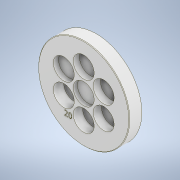
# Autodesk Inventor part: Diameter_20mm
Saved by Autodesk Inventor 2021 (Build 250183000, 183)
## iProperties
Created: 2023-09-28
Part Number: Diameter_20mm
Material: Polypropylen
Document SubType Name: Modeling
Designer: Konstantin
Density: 0.899 g/cm^3
Appearance: Glatt - Esche
Author: Konstantin
Autodesk Inventor part; units mm, degrees
ref_plane "YZ Plane" through (0, 0, 0) normal (1, 0, 0) x (0, 1, 0)
ref_plane "XZ Plane" through (0, 0, 0) normal (0, 1, 0) x (-1, 0, 0)
ref_plane "XY Plane" through (0, 0, 0) normal (0, 0, 1) x (1, 0, 0)
sketch "Sketch1" plane through (0, 0, 0) normal (0, 0, 1) x (1, 0, 0)
  circle A0 centre (0, 0) radius 43.5
  circle A1 centre (0, 0) radius 10
  circle A2 centre (0, 22) radius 10
  circle A3 centre (-19.0526, 11) radius 10
  circle A4 centre (-19.0526, -11) radius 10
  circle A5 centre (0, -22) radius 10
  circle A6 centre (19.0526, -11) radius 10
  circle A7 centre (19.0526, 11) radius 10
  dimension "diameter" = 20
  dimension "d2" = 20
  dimension "d5" = 360
  dimension "d7" = 22
  dimension "d28" = 87
  constraints: 8 centre point, 2 coincident, 13 other
  measures "diameter" diameter of A1
  measures "d2" diameter of A2
  measures "d7" distance of point (0, 0) A2.centre
  measures "d28" diameter of A0
extrude "Extrusion1" add sketch "Sketch1" along normal blind 12
sketch "Sketch2" plane through (0, 0, 12) normal (0, 0, 1) x (1, 0, 0)
  line L0 (-5.8774, 39.105) -> (5.7366, 39.105) construction
  line L1 (5.7366, 39.105) -> (5.7366, 35.936) construction
  line L2 (5.7366, 35.936) -> (-5.8774, 35.936) construction
  line L3 (-5.8774, 35.936) -> (-5.8774, 39.105) construction
  point P0 (0, 0)
  constraints: 2 other
emboss "Emboss1" [suppressed]
chamfer "Chamfer1" distance 0.5 angle 45 1 edges at (-43.5, 0, 12)
extrude "Extrusion11" add sketch "Sketch1" along normal blind 2 contours A4
extrude "Extrusion12" add sketch "Sketch1" along normal blind 3 contours A5
extrude "Extrusion13" add sketch "Sketch1" along normal blind 4 contours A6
extrude "Extrusion14" add sketch "Sketch1" along normal blind 5 contours A7
extrude "Extrusion15" add sketch "Sketch1" along normal blind 6 contours A2
extrude "Extrusion16" add sketch "Sketch1" along normal blind 7 contours A3
extrude "Extrusion17" add sketch "Sketch1" along normal blind 8 contours A1
sketch "Skizze3" plane through (0, 0, 12) normal (0, 0, 1) x (1, 0, 0)
  line L0 (-4.3129, -31.1582) -> (0.2616, -31.1582) construction
  line L1 (0.2616, -31.1582) -> (0.2616, -34.3322) construction
  line L2 (0.2616, -34.3322) -> (-4.3129, -34.3322) construction
  line L3 (-4.3129, -34.3322) -> (-4.3129, -31.1582) construction
  line L4 (28.3417, 16.1952) -> (30.6289, 16.1952) construction
  line L5 (30.6289, 16.1952) -> (30.6289, 13.0262) construction
  line L6 (30.6289, 13.0262) -> (28.3417, 13.0262) construction
  line L7 (28.3417, 13.0262) -> (28.3417, 16.1952) construction
  line L8 (-27.2854, 19.1878) -> (-24.9982, 19.1878) construction
  line L9 (-24.9982, 19.1878) -> (-24.9982, 16.0015) construction
  line L10 (-24.9982, 16.0015) -> (-27.2854, 16.0015) construction
  line L11 (-27.2854, 16.0015) -> (-27.2854, 19.1878) construction
  line L12 (-18.5838, -22.0358) -> (-14.0094, -22.0358) construction
  line L13 (-14.0094, -22.0358) -> (-14.0094, -25.2048) construction
  line L14 (-14.0094, -25.2048) -> (-18.5838, -25.2048) construction
  line L15 (-18.5838, -25.2048) -> (-18.5838, -22.0358) construction
  line L16 (-11.1833, -16.7575) -> (-8.896, -16.7575) construction
  line L17 (-8.896, -16.7575) -> (-8.896, -19.8055) construction
  line L18 (-8.896, -19.8055) -> (-11.1833, -19.8055) construction
  line L19 (-11.1833, -19.8055) -> (-11.1833, -16.7575) construction
  line L20 (20.4292, 1.4865) -> (22.7164, 1.4865) construction
  line L21 (22.7164, 1.4865) -> (22.7164, -1.6825) construction
  line L22 (22.7164, -1.6825) -> (20.4292, -1.6825) construction
  line L23 (20.4292, -1.6825) -> (20.4292, 1.4865) construction
  line L24 (-11.5764, 19.8878) -> (-9.2892, 19.8878) construction
  line L25 (-9.2892, 19.8878) -> (-9.2892, 16.7756) construction
  line L26 (-9.2892, 16.7756) -> (-11.5764, 16.7756) construction
  line L27 (-11.5764, 16.7756) -> (-11.5764, 19.8878) construction
  line L28 (3.9152, 10.1367) -> (6.2025, 10.1367) construction
  line L29 (6.2025, 10.1367) -> (6.2025, 7.0887) construction
  line L30 (6.2025, 7.0887) -> (3.9152, 7.0887) construction
  line L31 (3.9152, 7.0887) -> (3.9152, 10.1367) construction
  line L32 (-15.1357, -27.1411) -> (-18.2192, -27.1411)
  line L33 (-18.2192, -27.1411) -> (-18.2192, -26.432)
  spline S0 degree 2 poles (-18.2192, -26.432) (-17.8869, -26.12) (-17.2953, -25.5406) (-17.0117, -25.2286) knots 0 0 0 1 2 2 2
  spline S1 degree 2 poles (-17.0117, -25.2286) (-16.4404, -24.6006) (-16.023, -23.8469) (-16.023, -23.4458) knots 0 0 0 1 2 2 2
  spline S2 degree 2 poles (-16.023, -23.4458) (-16.023, -23.2351) (-16.1527, -22.9191) (-16.2702, -22.8178) knots 0 0 0 1 2 2 2
  spline S3 degree 2 poles (-16.2702, -22.8178) (-16.3877, -22.7165) (-16.6957, -22.6152) (-16.882, -22.6152) knots 0 0 0 1 2 2 2
  spline S4 degree 2 poles (-16.882, -22.6152) (-17.0603, -22.6152) (-17.425, -22.7043) (-17.5911, -22.7732) knots 0 0 0 1 2 2 2
  spline S5 degree 2 poles (-17.5911, -22.7732) (-17.7329, -22.8299) (-17.9963, -22.992) (-18.0773, -23.0487) knots 0 0 0 1 2 2 2
  line L34 (-18.0773, -23.0487) -> (-18.1138, -23.0487)
  line L35 (-18.1138, -23.0487) -> (-18.1138, -22.3356)
  spline S6 degree 2 poles (-18.1138, -22.3356) (-17.9072, -22.2343) (-17.1657, -22.0358) (-16.8334, -22.0358) knots 0 0 0 1 2 2 2
  spline S7 degree 2 poles (-16.8334, -22.0358) (-16.1324, -22.0358) (-15.3423, -22.7773) (-15.3423, -23.4093) knots 0 0 0 1 2 2 2
  spline S8 degree 2 poles (-15.3423, -23.4093) (-15.3423, -23.7051) (-15.4801, -24.1995) (-15.6017, -24.4102) knots 0 0 0 1 2 2 2
  spline S9 degree 2 poles (-15.6017, -24.4102) (-15.7232, -24.629) (-16.0757, -25.0585) (-16.2702, -25.2651) knots 0 0 0 1 2 2 2
  spline S10 degree 2 poles (-16.2702, -25.2651) (-16.5863, -25.6095) (-17.3602, -26.3469) (-17.5911, -26.5617) knots 0 0 0 1 2 2 2
  line L36 (-17.5911, -26.5617) -> (-15.1357, -26.5617)
  line L37 (-15.1357, -26.5617) -> (-15.1357, -27.1411)
  spline S11 degree 2 poles (-11.3553, -24.6411) (-11.3553, -25.9863) (-12.1373, -27.2465) (-12.9517, -27.2465) knots 0 0 0 1 2 2 2
  spline S12 degree 2 poles (-12.9517, -27.2465) (-13.7783, -27.2465) (-14.5522, -25.962) (-14.5522, -24.6452) knots 0 0 0 1 2 2 2
  spline S13 degree 2 poles (-14.5522, -24.6452) (-14.5522, -23.2918) (-13.7702, -22.0398) (-12.9517, -22.0398) knots 0 0 0 1 2 2 2
  spline S14 degree 2 poles (-12.9517, -22.0398) (-12.1292, -22.0398) (-11.3553, -23.3364) (-11.3553, -24.6411) knots 0 0 0 1 2 2 2
  spline S15 degree 2 poles (-12.2143, -26.1646) (-12.117, -25.9174) (-12.036, -25.1557) (-12.036, -24.6411) knots 0 0 0 1 2 2 2
  spline S16 degree 2 poles (-12.036, -24.6411) (-12.036, -24.1265) (-12.117, -23.3688) (-12.2183, -23.1136) knots 0 0 0 1 2 2 2
  spline S17 degree 2 poles (-12.2183, -23.1136) (-12.3196, -22.8583) (-12.6722, -22.5949) (-12.9517, -22.5949) knots 0 0 0 1 2 2 2
  spline S18 degree 2 poles (-12.9517, -22.5949) (-13.2313, -22.5949) (-13.5919, -22.8583) (-13.6973, -23.1217) knots 0 0 0 1 2 2 2
  spline S19 degree 2 poles (-13.6973, -23.1217) (-13.7986, -23.3769) (-13.8715, -24.1549) (-13.8715, -24.6452) knots 0 0 0 1 2 2 2
  spline S20 degree 2 poles (-13.8715, -24.6452) (-13.8715, -25.1719) (-13.8067, -25.8769) (-13.7013, -26.1525) knots 0 0 0 1 2 2 2
  spline S21 degree 2 poles (-13.7013, -26.1525) (-13.6041, -26.4118) (-13.2435, -26.6914) (-12.9517, -26.6914) knots 0 0 0 1 2 2 2
  spline S22 degree 2 poles (-12.9517, -26.6914) (-12.6762, -26.6914) (-12.3156, -26.428) (-12.2143, -26.1646) knots 0 0 0 1 2 2 2
  point P0 (0, 0)
  constraints: 16 other
emboss "Prägen2" sketch "Skizze3" operation cut depth 0.6 direction (0, 0, -1)
sketch "Skizze4" plane through (0, 0, 12) normal (0, 0, 1) x (1, 0, 0)
  circle A0 centre (0, 0) radius 40.5
  circle A1 centre (0, 0) radius 35
  dimension "d58" = 81
  dimension "d59" = 70
  constraints: 2 centre point, 2 coincident
  measures "d58" diameter of A0
  measures "d59" diameter of A1
extrude "Extrusion18" [suppressed]
equation "\"d2\" = diameter"
body "Solid1"
